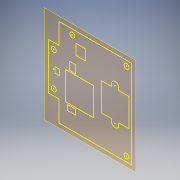
# Autodesk Inventor part: frontCase
Saved by Autodesk Inventor 2017 (Build 210142000, 142)
## iProperties
Created: 2016-12-21
Part Number: frontCase
Material: Generic
Document SubType Name: Modeling
Designer: PLTW
Density: 1 g/cm^3
Appearance: Default
Author: PLTW
Autodesk Inventor part; units mm, degrees
ref_plane "YZ Plane" through (0, 0, 0) normal (1, 0, 0) x (0, 1, 0)
ref_plane "XZ Plane" through (0, 0, 0) normal (0, 1, 0) x (-1, 0, 0)
ref_plane "XY Plane" through (0, 0, 0) normal (0, 0, 1) x (1, 0, 0)
ref_plane "Work Plane1" through (0, 0, 0) normal (0, 0, 1) x (1, 0, 0)
sketch "Sketch1" plane through (0, 0, 0) normal (0, 0, 1) x (1, 0, 0)
  line L0 (19.5326, 20.4724) -> (19.5326, 14.097) projected
  line L1 (19.5326, 14.097) -> (13.5636, 14.097) projected
  line L2 (13.5636, 14.097) -> (13.5636, 20.4724) projected
  line L3 (13.5636, 20.4724) -> (19.5326, 20.4724) projected
  line L4 (13.4112, 9.0424) -> (13.4112, 4.2164) projected
  line L5 (13.4112, 4.2164) -> (9.6012, 4.2164) projected
  line L6 (9.6012, 4.2164) -> (9.6012, 9.0424) projected
  line L7 (9.6012, 9.0424) -> (13.4112, 9.0424) projected
  line L8 (13.335, -14.5034) -> (13.335, -17.7038) projected
  line L9 (13.335, -17.7038) -> (8.3566, -17.7038) projected
  line L10 (8.3566, -17.7038) -> (8.3566, -14.5034) projected
  line L11 (8.3566, -14.5034) -> (13.335, -14.5034) projected
  line L12 (24.1808, 3.429) -> (24.1808, -13.589) projected
  line L13 (24.1808, -13.589) -> (7.1628, -13.589) projected
  line L14 (7.1628, -13.589) -> (7.1628, 3.429) projected
  line L15 (7.1628, 3.429) -> (24.1808, 3.429) projected
  line L16 (0.635, -1.7526) -> (0.635, 1.7526) projected
  line L17 (0.635, 1.7526) -> (3.4569, 1.7526) projected
  line L18 (3.4569, 1.7526) -> (3.4569, -1.7526) projected
  line L19 (3.4569, -1.7526) -> (0.635, -1.7526) projected
  arc A0 (35.2933, -10.0203) -> (39.7383, -10.0203) centre (37.5158, -10.0203) ccw projected
  line L20 (35.2933, -10.0203) -> (35.2933, -8.509) projected
  line L21 (35.2933, -8.509) -> (29.0068, -8.509) projected
  line L22 (29.0068, -8.509) -> (29.0068, 8.509) projected
  line L23 (29.0068, 8.509) -> (35.2933, 8.509) projected
  line L24 (35.2933, 8.509) -> (35.2933, 10.0203) projected
  arc A1 (39.7383, 10.0203) -> (35.2933, 10.0203) centre (37.5158, 10.0203) ccw projected
  line L25 (39.7383, 10.0203) -> (39.7383, 8.509) projected
  line L26 (39.7383, 8.509) -> (46.0248, 8.509) projected
  line L27 (46.0248, 8.509) -> (46.0248, -8.509) projected
  line L28 (46.0248, -8.509) -> (39.7383, -8.509) projected
  line L29 (39.7383, -8.509) -> (39.7383, -10.0203) projected
  circle A2 centre (11.303, 23.749) radius 1.524 projected
  circle A3 centre (44.45, -23.749) radius 1.524 projected
  circle A4 centre (44.45, 23.749) radius 1.524 projected
  circle A5 centre (0, -10.414) radius 1.524 projected
  circle A6 centre (0, 10.414) radius 1.524 projected
  line L30 (3.175, 14.224) -> (-3.175, 14.224) projected
  line L31 (-3.175, 14.224) -> (-3.175, -14.224) projected
  line L32 (-3.175, -14.224) -> (3.175, -14.224) projected
  line L33 (3.175, -14.224) -> (3.175, -26.924) projected
  line L34 (3.175, -26.924) -> (47.625, -26.924) projected
  line L35 (47.625, -26.924) -> (47.625, 26.924) projected
  line L36 (47.625, 26.924) -> (3.175, 26.924) projected
  line L37 (3.175, 26.924) -> (3.175, 14.224) projected
  circle A7 centre (44.45, -23.749) radius 1.524
  circle A8 centre (44.45, -23.749) radius 2.794
  circle A9 centre (44.45, 23.749) radius 1.524
  circle A10 centre (44.45, 23.749) radius 2.794
  point P0 (0, 0)
  dimension "d0" = 1.27
  constraints: 4 centre point, 4 coincident, 3 equal radius
  measures "d0" radial gap between concentric circles of A8 A3
ref_plane "Work Plane2" through (3.175, -9.6012, 2.286) normal (0, 0, 1) x (1, 0, 0)
extrude "Extrusion1" add sketch "Sketch1" along normal up to surface (2.286 mm away) contours A8 | A10
body "Solid1"
